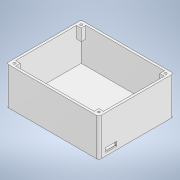
# Autodesk Inventor part: BH1750-case
Saved by Autodesk Inventor 2022 (Build 260153000, 153)
## iProperties
Created: 2023-05-13
Part Number: BH1750-case
Material: PVC potrubí
Document SubType Name: Modeling
Designer: tada
Density: 1.4 g/cm^3
Appearance: Hladká – bílá
Author: tada
Autodesk Inventor part; units mm, degrees
ref_plane "YZ Plane" through (0, 0, 0) normal (1, 0, 0) x (0, 1, 0)
ref_plane "XZ Plane" through (0, 0, 0) normal (0, 1, 0) x (-1, 0, 0)
ref_plane "XY Plane" through (0, 0, 0) normal (0, 0, 1) x (1, 0, 0)
sketch "Náčrt1" plane through (0, 0, 0) normal (0, 1, 0) x (-1, 0, 0)
  line L0 (0, 0) -> (-75, 0)
  line L1 (-75, 0) -> (-75, -60)
  line L2 (-75, -60) -> (0, -60)
  line L3 (0, -60) -> (0, 0)
  line L4 (2, 2) -> (-77, 2)
  line L5 (-77, 2) -> (-77, -62)
  line L6 (-77, -62) -> (2, -62)
  line L7 (2, -62) -> (2, 2)
  dimension "d0" = 60
  dimension "d1" = 75
  dimension "d2" = 2
  dimension "d3" = 2
  dimension "d4" = 2
  dimension "d5" = 2
  constraints: 16 end point, 4 parallel, 2 horizontal, 2 perpendicular
  measures "d0" distance of L2.end L0.start
  measures "d1" distance of L1.end L2.end
  measures "d2" distance between parallel lines of L7 L3
  measures "d3" distance between parallel lines of L6 L2
  measures "d4" distance between parallel lines of L1 L5
  measures "d5" distance between parallel lines of L4 L0
extrude "Vysunutí1" add sketch "Náčrt1" along normal blind 2 contours L3 L2 L1 L0
extrude "Vysunutí2" add sketch "Náčrt1" along normal blind 32
sketch "Náčrt2" plane through (0, 32, 0) normal (0, 1, 0) x (1, 0, 0)
  line L0 (-2, -2) -> (4, -2)
  line L1 (4, -2) -> (4, 4)
  line L2 (4, 4) -> (-2, 4)
  line L3 (-2, 4) -> (-2, -2)
  line L4 (77, 62) -> (-2, 62) projected
  line L5 (-2, 62) -> (4, 62)
  line L6 (4, 62) -> (4, 56)
  line L7 (4, 56) -> (-2, 56)
  line L8 (-2, 56) -> (-2, 62)
  line L9 (77, -2) -> (77, 62) projected
  line L10 (77, 62) -> (71, 62)
  line L11 (71, 62) -> (71, 56)
  line L12 (71, 56) -> (77, 56)
  line L13 (77, 56) -> (77, 62)
  line L14 (77, -2) -> (71, -2)
  line L15 (71, -2) -> (71, 4)
  line L16 (71, 4) -> (77, 4)
  line L17 (77, 4) -> (77, -2)
  point P0 (0, 0)
  dimension "d10" = 6
  dimension "d11" = 6
  dimension "d12" = 6
  dimension "d13" = 6
  dimension "d14" = 6
  dimension "d15" = 6
  dimension "d16" = 6
  dimension "d17" = 6
  constraints: 32 end point, 8 parallel, 4 horizontal, 4 perpendicular, 1 point on line
  measures "d10" distance of L2.end L0.start
  measures "d11" distance of L1.end L2.end
  measures "d12" distance of L4.end L5.end
  measures "d13" distance of L7.end L4.end
  measures "d14" distance of L10.end L11.end
  measures "d15" distance of L11.end L12.end
  measures "d16" distance of L14.end L15.end
  measures "d17" distance of L15.end L16.end
extrude "Vysunutí3" add sketch "Náčrt2" against normal blind 10
sketch "Náčrt3" plane through (0, 32, 0) normal (0, 1, 0) x (1, 0, 0)
  circle A0 centre (1.5, 58.5) radius 1
  line L0 (77, 62) -> (-2, 62) projected
  line L1 (-2, 62) -> (-2, -2) projected
  circle A1 centre (73.5, 58.5) radius 1
  line L2 (77, -2) -> (77, 62) projected
  circle A2 centre (73.5, 1.5) radius 1
  line L3 (-2, -2) -> (77, -2) projected
  circle A3 centre (1.5, 1.5) radius 1
  point P0 (0, 0)
  dimension "d20" = 2
  dimension "d21" = 3.5
  dimension "d22" = 3.5
  dimension "d23" = 2
  dimension "d24" = 3.5
  dimension "d25" = 3.5
  dimension "d26" = 2
  dimension "d27" = 3.5
  dimension "d28" = 3.5
  dimension "d29" = 2
  dimension "d30" = 3.5
  dimension "d31" = 3.5
  constraints: 4 centre point
  measures "d20" diameter of A0
  measures "d21" distance from line of L0 A0.centre
  measures "d22" distance from line of L1 A0.centre
  measures "d23" diameter of A1
  measures "d24" distance from line of L0 A1.centre
  measures "d25" distance from line of L2 A1.centre
  measures "d26" diameter of A2
  measures "d27" distance from line of L3 A2.centre
  measures "d28" distance from line of L2 A2.centre
  measures "d29" diameter of A3
  measures "d30" distance from line of L3 A3.centre
  measures "d31" distance from line of L1 A3.centre
extrude "Vysunutí4" cut sketch "Náčrt3" against normal blind 10 contours A0 | A1 | A2 | A3
sketch "Náčrt4" plane through (77, 0, 2) normal (1, 0, 0) x (0, 0, -1)
  line L0 (2, 2) -> (2, 22) projected
  line L1 (6.5, 5.7) -> (15, 5.7)
  line L2 (15, 5.7) -> (15, 3)
  line L3 (15, 3) -> (6.5, 3)
  line L4 (6.5, 3) -> (6.5, 5.7)
  line L5 (0, 0) -> (64, 0) projected
  point P0 (2, 0)
  dimension "d36" = 3
  dimension "d37" = 4.5
  dimension "d38" = 8.5
  dimension "d39" = 2.7
  constraints: 8 end point, 2 parallel, 1 horizontal, 1 perpendicular
  measures "d36" distance between parallel lines of L3 L5
  measures "d37" distance between parallel lines of L0 L4
  measures "d38" distance of L1.start L1.end
  measures "d39" distance between parallel lines of L1 L3
extrude "Vysunutí5" cut sketch "Náčrt4" against normal blind 10
sketch "Náčrt5" plane through (75, 2, -60) normal (-1, 0, 0) x (0, 0, 1)
  line L0 (60, 0) -> (0, 0) projected
  line L1 (42.65, 1) -> (60, 1)
  line L2 (60, 1) -> (60, 0)
  line L3 (60, 0) -> (42.65, 0)
  line L4 (42.65, 0) -> (42.65, 1)
  line L5 (60, 0) -> (60, 20) projected
  point P0 (60, -2)
  point P1 (60, 0.5)
  point P2 (42.65, 0)
  dimension "d42" = 17.35
  dimension "d43" = 1
  constraints: 8 end point, 2 parallel, 2 point on line, 1 horizontal, 1 midpoint, 1 perpendicular
  measures "d42" distance of L1.start L1.end
  measures "d43" distance of L3.end L1.start
extrude "Vysunutí6" cut sketch "Náčrt5" against normal blind 1
chamfer "Zkosení1" distance 0.5 angle 45 5 edges at (75.5, 3, -13) (75.5, 3, -4.5) (75, 4.35, -4.5) (75, 4.35, -13) (75, 5.7, -8.75)
chamfer "Zkosení2" distance 0.5 angle 45 4 edges at (77, 5.7, -8.75) (77, 4.35, -4.5) (77, 3, -8.75) (77, 4.35, -13)
sketch "Náčrt6" plane through (77, 0, 2) normal (1, 0, 0) x (0, 0, -1)
  point P0 (2, 0)
fillet "Zaoblení1" radius 2 4 edges at (77, 16, 2) (77, 16, -62) (-2, 16, -62) (-2, 16, 2)
equation "\"d3\" = d2"
equation "\"d4\" = d2"
equation "\"d5\" = d2"
equation "\"d12\" = d10"
equation "\"d13\" = d10"
equation "\"d14\" = d10"
equation "\"d15\" = d10"
equation "\"d16\" = d10"
equation "\"d23\" = d20"
equation "\"d24\" = d21"
equation "\"d25\" = d21"
equation "\"d26\" = d20"
equation "\"d27\" = d21"
equation "\"d28\" = d21"
equation "\"d29\" = d20"
equation "\"d30\" = d21"
equation "\"d31\" = d21"
